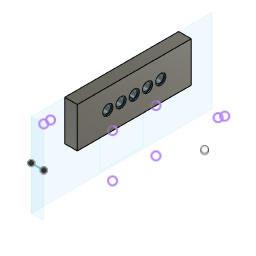
legotest v1 (Autodesk Fusion 360 design; units mm, degrees)
Autodesk Fusion 360 part; units mm, degrees
note: some values were not read from the file. Chosen so that the rebuilt part matches the saved one: which face or edge a step refers to; which pieces of a blend or face edit are solid. Set by a fixed rule: which sketch regions a step uses.
sketch "Sketch1" plane through (0, 0, 0) normal (0, 0, 1) x (1, 0, 0)
  line L0 (0, 0) -> (140, 0)
  line L1 (140, 0) -> (140, 150)
  line L2 (140, 150) -> (0, 150)
  line L3 (0, 150) -> (0, 0)
  constraint horizontal L0
  constraint vertical L1
  constraint horizontal L2
  constraint vertical L3
  constraint coincident L0.start L3.end
sketch "Sketch2" plane through (0, 0, 0) normal (0, 0, 1) x (1, 0, 0)
sketch "Sketch3" plane through (0, 0, 0) normal (0, 0, 1) x (1, 0, 0)
  line L0 (0, 0) -> (0, 100)
  line L1 (0, 100) -> (75, 100)
  line L2 (75, 100) -> (75, 0)
  line L3 (75, 0) -> (0, 0)
  line L4 (75, 100) -> (75, 104)
  line L5 (75, 104) -> (-7.5, 104)
  line L6 (-7.5, 104) -> (-7.5, -4)
  line L7 (-7.5, -4) -> (75, -4)
  line L8 (75, -4) -> (75, 0)
  dimension "d4" = 75
  dimension "d5" = 4
  dimension "d6" = 82.5
  dimension "d7" = 108
  dimension "d8" = 82.5
  constraint coincident L0.start L3.end
  constraint vertical L0
  constraint perpendicular L0 L1
  constraint perpendicular L1 L2
  constraint perpendicular L0 L3
  constraint perpendicular L1 L4
  constraint perpendicular L4 L5
  constraint perpendicular L5 L6
  constraint perpendicular L6 L7
  measures "d4" distance of L0.end L1.end
  measures "d5" distance of L1.end L4.end
  measures "d6" distance of L4.end L5.end
  measures "d7" distance of L5.end L6.end
  measures "d8" distance of L6.end L7.end
extrude "Extrude2" add sketch "Sketch3" along normal blind 50 contours L0 L1 L3 L4 L5 L6 L7 L8
sketch "Sketch4" plane through (0, 0, 0) normal (0, 0, 1) x (1, 0, 0)
sketch "Sketch5" plane through (0, 0, 0) normal (0, 0, 1) x (1, 0, 0)
  line L0 (75, 0) -> (75, 100)
  line L1 (75, 100) -> (0, 100)
  line L2 (0, 100) -> (0, 0)
  line L3 (0, 0) -> (75, 0)
  constraint vertical L0
  constraint perpendicular L0 L1
  constraint coincident L2.end L3.start
  constraint perpendicular L1 L2
  constraint perpendicular L0 L3
extrude "Extrude3" add sketch "Sketch5" along normal blind 1.2
sketch "Sketch6" plane through (0, 0, 0) normal (1, 0, 0) x (0, 1, 0)
  line L0 (100, 1.2) -> (100, 50)
  line L1 (100, 50) -> (0, 50)
sketch "Sketch7" plane through (0, 0, 0) normal (1, 0, 0) x (0, 1, 0)
  line L0 (92, -12) -> (91.9892, -11.1216)
sketch "Sketch8" plane through (0, 0, 0) normal (1, 0, 0) x (0, 1, 0)
sketch "Sketch9" plane through (0, 0, 0) normal (1, 0, 0) x (0, 1, 0)
sketch "Sketch10" plane through (0, 0, 0) normal (1, 0, 0) x (0, 1, 0)
  line L0 (0, 1.2) -> (100, 1.2)
  line L1 (100, 1.2) -> (100, 50)
  line L2 (100, 50) -> (0, 50)
  line L3 (0, 50) -> (0, 1.2)
  line L4 (37.0644, 1.2) -> (37.0644, 26)
  line L5 (37.0644, 26) -> (50, 26)
  line L6 (7, 61) -> (6, 65)
  line L7 (62.9356, 26) -> (50, 26)
  line L8 (62.9356, 1.2) -> (62.9356, 26)
  constraint coincident L0 L4.start
  constraint perpendicular L0 L4
  constraint perpendicular L4 L5
  constraint horizontal L7
  constraint vertical L8
sketch "Sketch11" plane through (0, 0, 0) normal (1, 0, 0) x (0, 1, 0)
extrude "Extrude4" cut sketch "Sketch10" against normal blind 16 contours L0 L4 L5 L7 L8
sketch "Sketch12" plane through (0, 0, 0) normal (1, 0, 0) x (0, 1, 0)
sketch "Sketch19" plane through (-7.5, 0, 0) normal (-1, 0, 0) x (0, -1, 0)
  line L0 (-62.9356, 1.2) -> (-62.9356, 26)
  line L1 (-62.9356, 26) -> (-37.0644, 26)
  line L2 (-37.0644, 26) -> (-37.0644, 1.2)
  line L3 (-37.0644, 1.2) -> (-62.9356, 1.2)
  line L4 (-104, 0) -> (4, 0)
  line L5 (4, 0) -> (4, 50)
  line L6 (4, 50) -> (-104, 50)
  line L7 (-104, 50) -> (-104, 0)
  line L8 (-50, 26) -> (-50, 50)
  circle A0 centre (-50, 38) radius 3.05
  line L9 (-53.0499, 38.0261) -> (-54.8499, 38.0261)
  circle A1 centre (-57.8999, 38.0261) radius 3.05
  line L10 (-60.9495, 37.9796) -> (-62.7495, 37.9796)
  circle A2 centre (-65.7995, 37.9942) radius 3.05
  circle A3 centre (-34.2005, 37.9942) radius 3.05
  circle A4 centre (-42.1001, 38.0261) radius 3.05
  line L11 (-46.9501, 38.0261) -> (-45.1501, 38.0261)
  line L12 (-39.0505, 37.9796) -> (-37.2505, 37.9796)
  circle A5 centre (-50, 38) radius 2.35
  circle A6 centre (-65.7995, 37.9942) radius 2.35
  circle A7 centre (-57.8999, 38.0261) radius 2.35
  circle A8 centre (-42.1001, 38.0261) radius 2.35
  circle A9 centre (-34.2005, 37.9942) radius 2.35
  dimension "d35" = 6.1
  dimension "d36" = 1.8
  dimension "d37" = 6.1
  dimension "d38" = 1.8
  dimension "d39" = 6.1
  dimension "d40" = 4.7
  dimension "d41" = 4.7
  dimension "d42" = 4.7
  dimension "d43" = 4.7
  dimension "d44" = 4.7
  constraint midpoint L1 L8.start
  constraint midpoint L6 L8.end
  constraint midpoint L8 A0.centre
  constraint coincident A0 L9.start
  constraint horizontal L9
  constraint coincident L9.end A1
  constraint coincident A1 L10.start
  constraint horizontal L10
  constraint coincident L10.end A2
  constraint symmetric L8 L9.start L11.start
  constraint symmetric L8 L9.end L11.end
  constraint symmetric L8 A1 A4
  constraint symmetric L8 L10.start L12.start
  constraint symmetric L8 L10.end L12.end
  constraint symmetric L8 A2 A3
  constraint concentric A0 A5
  constraint concentric A2 A6
  constraint concentric A1 A7
  constraint concentric A4 A8
  constraint concentric A3 A9
  measures "d35" diameter of A0
  measures "d36" distance of L9.start L9.end
  measures "d37" diameter of A1
  measures "d38" distance of L10.start L10.end
  measures "d39" diameter of A2
  measures "d40" diameter of A5
  measures "d41" diameter of A6
  measures "d42" diameter of A7
  measures "d43" diameter of A8
  measures "d44" diameter of A9
sketch "Sketch13" plane through (-7.5, 0, 0) normal (-1, 0, 0) x (0, -1, 0)
  line L0 (-62.9356, 1.2) -> (-62.9356, 26)
  line L1 (-62.9356, 26) -> (-37.0644, 26)
  line L2 (-37.0644, 26) -> (-37.0644, 1.2)
  line L3 (-37.0644, 1.2) -> (-62.9356, 1.2)
  line L4 (-104, 0) -> (4, 0)
  line L5 (4, 0) -> (4, 50)
  line L6 (4, 50) -> (-104, 50)
  line L7 (-104, 50) -> (-104, 0)
sketch "Sketch14" plane through (-7.5, 50, 25) normal (-1, 0, 0) x (0, -1, 0)
  line L0 (0.0006, 25) -> (0.0006, 1)
  line L1 (-12.9356, 1) -> (12.9356, 1)
  line L2 (54, 25) -> (-54, 25)
  circle A0 centre (0.0006, 13) radius 3.05
  circle A1 centre (0.0006, 13) radius 2.35
  dimension "d18" = 6.1
  dimension "d19" = 4.7
  constraint vertical L0
  constraint coincident L0.end L1
  constraint coincident L0.start L2
  constraint midpoint L0 A0.centre
  constraint concentric A0 A1
  measures "d18" diameter of A0
  measures "d19" diameter of A1
sketch "Sketch15" plane through (-7.5, 50, 25) normal (-1, 0, 0) x (0, -1, 0)
sketch "Sketch16" plane through (-7.5, 0, 0) normal (-1, 0, 0) x (0, -1, 0)
  line L0 (-53.0494, 38) -> (-54.8494, 38)
  circle A0 centre (-57.8994, 38) radius 3.05
  circle A1 centre (-57.8994, 38) radius 2.35
  circle A2 centre (-49.9994, 38) radius 3.05
  line L1 (-60.9494, 38) -> (-62.7494, 38)
  circle A3 centre (-65.8, 38.1) radius 3.05
  circle A4 centre (-65.8, 38.1) radius 2.35
  line L2 (-49.9994, 50) -> (-49.9994, 26)
  circle A5 centre (-42.0994, 38) radius 2.35
  circle A6 centre (-42.0994, 38) radius 3.05
  circle A7 centre (-34.1988, 38.1) radius 2.35
  circle A8 centre (-34.1988, 38.1) radius 3.05
  line L3 (-39.0494, 38) -> (-37.2494, 38)
  line L4 (-46.9494, 38) -> (-45.1494, 38)
  dimension "d24" = 1.8
  dimension "d25" = 6.1
  dimension "d26" = 4.7
  dimension "d27" = 1.8
  dimension "d28" = 6.1
  dimension "d29" = 4.7
  constraint horizontal L0
  constraint concentric A0 A1
  constraint coincident L0.end A0
  constraint coincident L0.start A2
  constraint horizontal L1
  constraint coincident A0 L1.start
  constraint concentric A3 A4
  constraint symmetric L0.start L2 L4.start
  constraint symmetric L0.end L2 L4.end
  constraint symmetric A0 L2 A6
  constraint symmetric A1 L2 A5
  constraint symmetric L1.start L2 L3.start
  constraint symmetric L1.end L2 L3.end
  constraint symmetric A3 L2 A8
  constraint symmetric A4 L2 A7
  measures "d24" distance of L0.start L0.end
  measures "d25" diameter of A0
  measures "d26" diameter of A1
  measures "d27" distance of L1.start L1.end
  measures "d28" diameter of A3
  measures "d29" diameter of A4
extrude "Extrude5" cut sketch "Sketch16" against normal blind 19 contours A4
sketch "Sketch18" plane through (-7.5, 50, 25) normal (-1, 0, 0) x (0, -1, 0)
sketch "Sketch17" plane through (-7.5, 0, 0) normal (-1, 0, 0) x (0, -1, 0)
extrude "Extrude6" cut sketch "Sketch14" against normal blind 7 contours L0 A1 picked at (0.839, 13.6628)
hole "Hole1" at (-7.5, 57.8999, 38.0261) direction (1, 0, 0) diameter 4.7 depth 8 tip angle 180
sketch "Sketch20" plane through (-7.5, 0, 0) normal (-1, 0, 0) x (0, -1, 0)
sketch "Sketch21" plane through (-7.5, 0, 0) normal (-1, 0, 0) x (0, -1, 0)
  line L0 (-50, 50) -> (-50, 26)
  circle A0 centre (-50, 38) radius 3.05
  circle A1 centre (-57.8999, 38.0261) radius 3.05
  circle A2 centre (-57.8999, 38.0261) radius 2.35
  circle A3 centre (-65.8, 38.1) radius 2.9921
  circle A4 centre (-65.8, 38.1) radius 2.35
  circle A5 centre (-50, 38) radius 2.35
  dimension "d48" = 6.1
  dimension "d49" = 6.1
  dimension "d50" = 4.7
  constraint vertical L0
  constraint midpoint L0 A0.centre
  constraint concentric A1 A2
  constraint concentric A3 A4
  constraint concentric A0 A5
  measures "d48" diameter of A0
  measures "d49" diameter of A1
  measures "d50" diameter of A5
hole "Hole2" at (-7.5, 50, 38) direction (1, 0, 0) diameter 4.7 depth 8 tip angle 180
sketch "Sketch22" plane through (-7.5, 0, 0) normal (-1, 0, 0) x (0, -1, 0)
  line L0 (-50, 50) -> (-50, 26)
  circle A0 centre (-65.8, 38.1) radius 2.35
  circle A1 centre (-65.8, 38.1) radius 2.35
  circle A2 centre (-34.2, 38.1) radius 2.35
  dimension "d54" = 4.7
  constraint vertical L0
  constraint concentric A0 A1
  constraint symmetric L0 A0 A2
  measures "d54" diameter of A0
hole "Hole3" at (-7.5, 34.2, 38.1) direction (1, 0, 0) diameter 4.7 depth 8 tip angle 180
sketch "Sketch23" plane through (-7.5, 0, 0) normal (-1, 0, 0) x (0, -1, 0)
  circle A0 centre (-57.8999, 38.0261) radius 2.35
  circle A1 centre (-57.8999, 38.0261) radius 2.35
  line L0 (-50, 50) -> (-50, 26)
  circle A2 centre (-42.1001, 38.0261) radius 2.35
  dimension "d58" = 4.7
  constraint concentric A0 A1
  constraint vertical L0
  constraint symmetric A0 L0 A2
  measures "d58" diameter of A0
hole "Hole4" at (-7.5, 42.1001, 38.0261) direction (1, 0, 0) diameter 4.7 depth 8 tip angle 180
sketch "Sketch24" plane through (-7.5, 0, 0) normal (-1, 0, 0) x (0, -1, 0)
  circle A0 centre (-65.8, 38.1) radius 3.05
  circle A1 centre (-65.8, 38.1) radius 2.35
  dimension "d62" = 6.1
  constraint concentric A0 A1
  measures "d62" diameter of A0
sketch "Sketch25" plane through (-7.5, 0, 0) normal (-1, 0, 0) x (0, -1, 0)
  circle A0 centre (-65.8, 38.1) radius 3.05
  circle A1 centre (-65.8, 38.1) radius 2.35
  dimension "d66" = 6.1
  constraint concentric A0 A1
  measures "d66" diameter of A0
sketch "Sketch26" plane through (-7.5, 0, 0) normal (-1, 0, 0) x (0, -1, 0)
  circle A0 centre (-65.8, 38.1) radius 3.05
  circle A1 centre (-65.8, 38.1) radius 2.35
  dimension "d70" = 6.1
  constraint concentric A0 A1
  measures "d70" diameter of A0
sketch "Sketch27" plane through (-7.5, 0, 0) normal (-1, 0, 0) x (0, -1, 0)
  circle A0 centre (-65.8, 38.1) radius 3.05
  circle A1 centre (-65.8, 38.1) radius 2.35
  dimension "d74" = 6.1
  constraint concentric A0 A1
  measures "d74" diameter of A0
hole "Hole8" at (-7.5, 65.8, 38.1) direction (1, 0, 0) diameter 6.1 depth 0.7 tip angle 180
sketch "Sketch28" plane through (-7.5, 0, 0) normal (-1, 0, 0) x (0, -1, 0)
  circle A0 centre (-58, 38) radius 3.05
  dimension "d78" = 6.1
  measures "d78" diameter of A0
sketch "Sketch29" plane through (-7.5, 0, 0) normal (-1, 0, 0) x (0, -1, 0)
  circle A0 centre (-57.8999, 38.0261) radius 3.05
  circle A1 centre (-57.8999, 38.0261) radius 2.35
  dimension "d82" = 6.1
  constraint concentric A0 A1
  measures "d82" diameter of A0
hole "Hole10" at (-7.5, 57.8999, 38.0261) direction (1, 0, 0) diameter 6.1 depth 0.7 tip angle 180
sketch "Sketch30" plane through (-7.5, 0, 0) normal (-1, 0, 0) x (0, -1, 0)
  circle A0 centre (-50, 38) radius 3.05
  dimension "d86" = 6.1
  measures "d86" diameter of A0
hole "Hole11" at (-7.5, 50, 38) direction (1, 0, 0) diameter 6.1 depth 0.7 tip angle 180
sketch "Sketch31" plane through (-7.5, 0, 0) normal (-1, 0, 0) x (0, -1, 0)
  circle A0 centre (-42.1001, 38.0261) radius 3.05
  circle A1 centre (-42.1001, 38.0261) radius 2.35
  dimension "d90" = 6.1
  constraint concentric A0 A1
  measures "d90" diameter of A0
hole "Hole12" at (-7.5, 42.1001, 38.0261) direction (1, 0, 0) diameter 6.1 depth 0.7 tip angle 180
sketch "Sketch32" plane through (-7.5, 0, 0) normal (-1, 0, 0) x (0, -1, 0)
  circle A0 centre (-34.2, 38.1) radius 3.05
  circle A1 centre (-34.2, 38.1) radius 2.35
  dimension "d94" = 6.1
  constraint concentric A0 A1
  measures "d94" diameter of A0
hole "Hole13" at (-7.5, 34.2, 38.1) direction (1, 0, 0) diameter 6.1 depth 0.7 tip angle 180
sketch "Sketch33" plane through (0, 0, 0) normal (1, 0, 0) x (0, 1, 0)
  circle A0 centre (34.2, 38.1) radius 3.05
  circle A1 centre (34.2, 38.1) radius 2.35
  dimension "d98" = 6.1
  constraint concentric A0 A1
  measures "d98" diameter of A0
hole "Hole14" at (0, 34.2, 38.1) direction (-1, 0, 0) diameter 6.1 depth 0.7 tip angle 180
sketch "Sketch34" plane through (0, 0, 0) normal (1, 0, 0) x (0, 1, 0)
  circle A0 centre (42.1001, 38.0261) radius 3.05
  circle A1 centre (42.1001, 38.0261) radius 2.35
  dimension "d102" = 6.1
  constraint concentric A0 A1
  measures "d102" diameter of A0
hole "Hole15" at (0, 42.1001, 38.0261) direction (-1, 0, 0) diameter 6.1 depth 0.7 tip angle 180
sketch "Sketch35" plane through (0, 0, 0) normal (1, 0, 0) x (0, 1, 0)
  circle A0 centre (50, 38) radius 3.05
  dimension "d107" = 6.1
  measures "d107" diameter of A0
hole "Hole16" at (0, 50, 38) direction (-1, 0, 0) diameter 6.1 depth 0.7 tip angle 180
sketch "Sketch36" plane through (0, 0, 0) normal (1, 0, 0) x (0, 1, 0)
  circle A0 centre (57.8999, 38.0261) radius 3.05
  circle A1 centre (57.8999, 38.0261) radius 2.35
  dimension "d111" = 6.1
  constraint concentric A0 A1
  measures "d111" diameter of A0
hole "Hole17" at (0, 57.8999, 38.0261) direction (-1, 0, 0) diameter 6.1 depth 0.7 tip angle 180
sketch "Sketch37" plane through (0, 0, 0) normal (1, 0, 0) x (0, 1, 0)
  circle A0 centre (65.8, 38.1) radius 3.05
  circle A1 centre (65.8, 38.1) radius 2.35
  dimension "d115" = 6.1
  constraint concentric A0 A1
  measures "d115" diameter of A0
hole "Hole18" at (0, 65.8, 38.1) direction (-1, 0, 0) diameter 6.1 depth 0.7 tip angle 180
delete_face "DeleteFace1" 1 faces at (50, 45.6881, 1.2)
extrude "Extrude7" cut 1 faces at (75, -2.6667, 16.6667) along direction (-1, 0, 0) blind 75
extrude "Extrude8" cut 1 faces at (75, 101.3333, 16.6667) along direction (-1, 0, 0) blind 75
sketch "Sketch38" plane through (0, 0, 0) normal (1, 0, 0) x (0, 1, 0)
  line L0 (37.0644, 26) -> (62.9356, 26)
  line L1 (62.9356, 0) -> (104, 0)
  line L2 (-4, 50) -> (-4, 0)
  line L3 (-4, 0) -> (37.0644, 0)
  circle A0 centre (65.8, 38.1) radius 3.05
  circle A1 centre (57.8999, 38.0261) radius 3.05
  circle A2 centre (50, 38) radius 3.05
  circle A3 centre (42.1001, 38.0261) radius 3.05
  circle A4 centre (34.2, 38.1) radius 3.05
delete_face "DeleteFace2" 3 faces at (-5, 76.6238, 0) (-5, 62.9356, 8.6667) (-2.5, 104, 16.6667)
sketch "Sketch39" plane through (0, 0, 0) normal (0, 1, 0) x (1, 0, 0)
sketch "Sketch40" plane through (0, -4, 0) normal (0, -1, 0) x (1, 0, 0)
  line L0 (0, 0) -> (0, 50)
  line L1 (0, 50) -> (-7.5, 50)
  line L2 (-7.5, 50) -> (-7.5, 0)
  line L3 (-7.5, 0) -> (0, 0)
  line L4 (0, 26) -> (-7.5, 26)
  constraint coincident L0 L4.start
  constraint coincident L2 L4.end
  constraint perpendicular L2 L4
extrude "Extrude9" cut 1 faces at (-5, 9.6881, 0) along direction (0, 0, 1) blind 26
extrude "Extrude10" cut 1 faces at (-2.5, -4, 42) along direction (0, 1, 0) blind 20
extrude "Extrude11" cut 1 faces at (-2.5, 104, 34) along direction (0, -1, 0) blind 20
hole "Hole9" [suppressed]
hole "Hole7" [suppressed]
hole "Hole6" [suppressed]
hole "Hole5" [suppressed]
